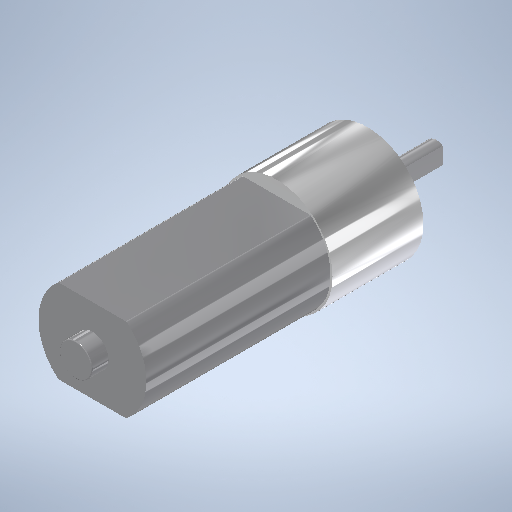
# Autodesk Inventor part: Dc Motor 3mm D Shaft
Saved by Autodesk Inventor 2025.3 (Build 293356000, 356)
## iProperties
Created: 2017-08-30
Part Number: Dc Motor 3mm D Shaft
Material: Generic
Document SubType Name: Modeling
Designer: PARAMA DIPTYA W
Density: 1 g/cm^3
Appearance: Default
Author: PARAMA DIPTYA W
Autodesk Inventor part; units mm, degrees
ref_plane "YZ Plane" through (0, 0, 0) normal (1, 0, 0) x (0, 1, 0)
ref_plane "XZ Plane" through (0, 0, 0) normal (0, 1, 0) x (-1, 0, 0)
ref_plane "XY Plane" through (0, 0, 0) normal (0, 0, 1) x (1, 0, 0)
sketch "Sketch1" plane through (0, 0, 0) normal (0, 1, 0) x (-1, 0, 0)
  circle A0 centre (0, 0) radius 8
  dimension "d0" = 16
  constraints: 1 centre point, 1 coincident
  measures "d0" diameter of A0
extrude "Extrusion1" add sketch "Sketch1" along normal blind 13
sketch "Sketch2" plane through (0, 13, 0) normal (0, 1, 0) x (1, 0, 0)
  circle A0 centre (0, 0) radius 3
  dimension "d3" = 6
  constraints: 1 centre point, 1 coincident
  measures "d3" diameter of A0
extrude "Extrusion2" add sketch "Sketch2" along normal blind 1.85
sketch "Sketch3" plane through (0, 14.85, 0) normal (0, 1, 0) x (1, 0, 0)
  circle A0 centre (0, 0) radius 1.5
  dimension "d6" = 3
  constraints: 1 centre point, 1 coincident
  measures "d6" diameter of A0
extrude "Extrusion3" add sketch "Sketch3" along normal blind 8
sketch "Sketch4" plane through (0, 22.85, 0) normal (0, 1, 0) x (1, 0, 0)
  circle A0 centre (0, 0) radius 1.5 projected
  line L0 (0.9, 0) -> (0.9, 1.2)
  line L1 (0.9, 1.2) -> (0.9, -1.2)
  circle A1 centre (0, 0) radius 3 projected
  arc A2 (0.9, -1.2) -> (0.9, 1.2) centre (0, 0) ccw
  constraints: 4 end point, 4 point on circle, 1 centre point, 1 coincident, 1 concentric, 1 point on line
extrude "Extrusion4" cut sketch "Sketch4" against normal blind 7 contours A0 L1 L0 picked at (0.9839, 0.7204)
sketch "Sketch5" plane through (0, 13, 0) normal (0, 1, 0) x (1, 0, 0)
  circle A0 centre (5, 0) radius 1.5
  circle A1 centre (-5, 0) radius 1.5
  point P0 (0, 0)
  constraints: 2 centre point
extrude "Extrusion5" cut sketch "Sketch5" against normal blind 2
sketch "Sketch6" plane through (0, 13, 0) normal (0, 1, 0) x (1, 0, 0)
  circle A0 centre (0, 0) radius 8 projected
  circle A1 centre (0, -5.45) radius 0.775
  line L0 (-8, 0) -> (8, 0)
  circle A2 centre (0, 5.45) radius 0.775
  constraints: 2 centre point, 2 end point, 2 point on circle, 1 horizontal, 1 symmetric about line, 1 other
extrude "Extrusion6" cut sketch "Sketch6" against normal blind 2 contours A1 | A2
sketch "Sketch7" plane through (0, 13, 0) normal (0, 1, 0) x (1, 0, 0)
  point P0 (0, 0)
sketch "Sketch8" plane through (0, 0, 0) normal (0, -1, 0) x (1, 0, 0)
  circle A0 centre (0, 0) radius 7.725
  dimension "d22" = 15.45
  constraints: 1 centre point, 1 coincident
  measures "d22" diameter of A0
extrude "Extrusion7" add sketch "Sketch8" along normal blind 26.35
sketch "Sketch9" plane through (0, -26.35, 0) normal (0, -1, 0) x (1, 0, 0)
  line L0 (0, -6) -> (-4.8658, -6)
  circle A0 centre (0, 0) radius 7.725 projected
  line L1 (0, -6) -> (4.8658, -6)
  line L2 (0, 6) -> (-4.8653, 6.0004)
  line L3 (0, 6) -> (4.8652, 6.0004)
  arc A1 (-4.8658, -6) -> (4.8658, -6) centre (0, 0) ccw
  arc A2 (4.8652, 6.0004) -> (-4.8653, 6.0004) centre (0, 0) ccw
  constraints: 8 end point, 8 point on circle, 2 centre point, 1 coincident, 1 horizontal, 1 point on line
extrude "Extrusion8" cut sketch "Sketch9" against normal blind 26.35 contours L1 A0 L0 | A0 L3 L2
sketch "Sketch10" plane through (0, -26.35, 0) normal (0, -1, 0) x (1, 0, 0)
  circle A0 centre (0, 0) radius 2.325
  dimension "d29" = 4.65
  constraints: 1 centre point, 1 coincident
  measures "d29" diameter of A0
extrude "Extrusion9" add sketch "Sketch10" along normal blind 2.4
fillet "Fillet1" radius 0.125 1 edges at (-2.325, -28.75, 0)
fillet "Fillet2" radius 0.05 1 edges at (-3, 14.85, 0)
fillet "Fillet3" radius 0.25 4 edges at (-4.8658, -13.175, -6) (4.8658, -13.175, -6) (-4.8653, -13.175, 6.0004) (4.8652, -13.175, 6.0004)
body "Solid1"
